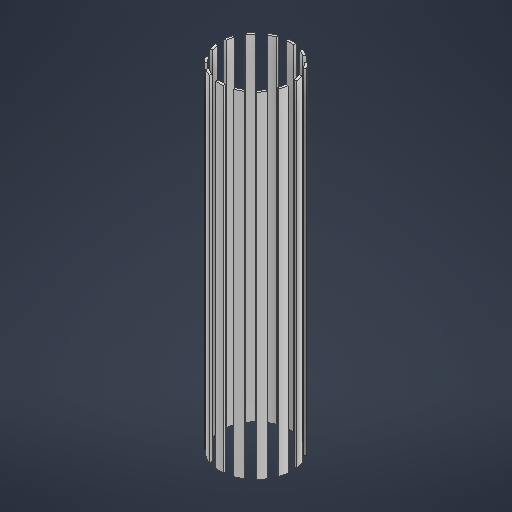
# Autodesk Inventor part: bandspreroller
Saved by Autodesk Inventor 2026.1 (Build 301233000, 233)
## iProperties
Created: 2025-08-08
Part Number: bandspreroller
Material: Generic
Document SubType Name: Modeling
Designer: roejo
Density: 1 g/cm^3
Appearance: Default
Author: roejo
Autodesk Inventor part; units mm, degrees
ref_plane "YZ Plane" through (0, 0, 0) normal (1, 0, 0) x (0, 1, 0)
ref_plane "XZ Plane" through (0, 0, 0) normal (0, 1, 0) x (-1, 0, 0)
ref_plane "XY Plane" through (0, 0, 0) normal (0, 0, 1) x (1, 0, 0)
sketch "Sketch1" plane through (0, 0, 0) normal (0, 1, 0) x (-1, 0, 0)
  circle A0 centre (0, 0) radius 24.4475
  dimension "d0" = 48.895
  constraints: 1 centre point, 1 coincident
  measures "d0" diameter of A0
extrude "Extrusion1" add sketch "Sketch1" along normal blind 224.3328
sketch "Sketch2" plane through (0, 224.3328, 0) normal (0, 1, 0) x (1, 0, 0)
  circle A0 centre (0, 0) radius 22.86
  dimension "d3" = 45.72
  constraints: 1 centre point, 1 coincident
  measures "d3" diameter of A0
extrude "Extrusion2" cut sketch "Sketch2" against normal through all
sketch "Sketch3" plane through (0, 224.3328, 0) normal (0, 1, 0) x (1, 0, 0)
  line L0 (-25.4, -2.8575) -> (-12.7, -2.8575)
  line L1 (-12.7, -2.8575) -> (-12.7, 2.8575)
  line L2 (-12.7, 2.8575) -> (-25.4, 2.8575)
  line L3 (-25.4, 2.8575) -> (-25.4, -2.8575)
  line L4 (-21.6448, -13.5952) -> (-10.2025, -8.0848)
  line L5 (-10.2025, -8.0848) -> (-12.6821, -2.9358)
  line L6 (-12.6821, -2.9358) -> (-24.1244, -8.4461)
  line L7 (-24.1244, -8.4461) -> (-21.6448, -13.5952)
  line L8 (-13.6026, -21.6401) -> (-5.6842, -11.7109)
  line L9 (-5.6842, -11.7109) -> (-10.1524, -8.1476)
  line L10 (-10.1524, -8.1476) -> (-18.0707, -18.0769)
  line L11 (-18.0707, -18.0769) -> (-13.6026, -21.6401)
  line L12 (-2.8662, -25.399) -> (-0.0402, -13.0174)
  line L13 (-0.0402, -13.0174) -> (-5.6119, -11.7457)
  line L14 (-5.6119, -11.7457) -> (-8.4379, -24.1273)
  line L15 (-8.4379, -24.1273) -> (-2.8662, -25.399)
  line L16 (8.4379, -24.1273) -> (5.6119, -11.7457)
  line L17 (5.6119, -11.7457) -> (0.0402, -13.0174)
  line L18 (0.0402, -13.0174) -> (2.8662, -25.399)
  line L19 (2.8662, -25.399) -> (8.4379, -24.1273)
  line L20 (18.0707, -18.0769) -> (10.1524, -8.1476)
  line L21 (10.1524, -8.1476) -> (5.6842, -11.7109)
  line L22 (5.6842, -11.7109) -> (13.6026, -21.6401)
  line L23 (13.6026, -21.6401) -> (18.0707, -18.0769)
  line L24 (24.1244, -8.4461) -> (12.6821, -2.9358)
  line L25 (12.6821, -2.9358) -> (10.2025, -8.0848)
  line L26 (10.2025, -8.0848) -> (21.6448, -13.5952)
  line L27 (21.6448, -13.5952) -> (24.1244, -8.4461)
  line L28 (25.4, 2.8575) -> (12.7, 2.8575)
  line L29 (12.7, 2.8575) -> (12.7, -2.8575)
  line L30 (12.7, -2.8575) -> (25.4, -2.8575)
  line L31 (25.4, -2.8575) -> (25.4, 2.8575)
  circle A0 centre (0, 0) radius 24.4475 projected
  line L32 (21.6448, 13.5952) -> (10.2025, 8.0848)
  line L33 (10.2025, 8.0848) -> (12.6821, 2.9358)
  line L34 (12.6821, 2.9358) -> (24.1244, 8.4461)
  line L35 (24.1244, 8.4461) -> (21.6448, 13.5952)
  line L36 (13.6026, 21.6401) -> (5.6842, 11.7109)
  line L37 (5.6842, 11.7109) -> (10.1524, 8.1476)
  line L38 (10.1524, 8.1476) -> (18.0707, 18.0769)
  line L39 (18.0707, 18.0769) -> (13.6026, 21.6401)
  line L40 (2.8662, 25.399) -> (0.0402, 13.0174)
  line L41 (0.0402, 13.0174) -> (5.6119, 11.7457)
  line L42 (5.6119, 11.7457) -> (8.4379, 24.1273)
  line L43 (8.4379, 24.1273) -> (2.8662, 25.399)
  line L44 (-8.4379, 24.1273) -> (-5.6119, 11.7457)
  line L45 (-5.6119, 11.7457) -> (-0.0402, 13.0174)
  line L46 (-0.0402, 13.0174) -> (-2.8662, 25.399)
  line L47 (-2.8662, 25.399) -> (-8.4379, 24.1273)
  line L48 (-18.0707, 18.0769) -> (-10.1524, 8.1476)
  line L49 (-10.1524, 8.1476) -> (-5.6842, 11.7109)
  line L50 (-5.6842, 11.7109) -> (-13.6026, 21.6401)
  line L51 (-13.6026, 21.6401) -> (-18.0707, 18.0769)
  line L52 (-24.1244, 8.4461) -> (-12.6821, 2.9358)
  line L53 (-12.6821, 2.9358) -> (-10.2025, 8.0848)
  line L54 (-10.2025, 8.0848) -> (-21.6448, 13.5952)
  line L55 (-21.6448, 13.5952) -> (-24.1244, 8.4461)
  point P0 (-30.1625, 0)
  point P1 (-27.1755, -13.087)
  point P2 (-18.806, -23.582)
  point P3 (-6.7118, -29.4063)
  point P4 (6.7118, -29.4063)
  point P5 (18.806, -23.582)
  point P6 (27.1755, -13.087)
  point P7 (30.1625, 0)
  point P8 (27.1755, 13.087)
  point P9 (18.806, 23.582)
  point P10 (6.7118, 29.4063)
  point P11 (-6.7118, 29.4063)
  point P12 (-18.806, 23.582)
  point P13 (-27.1755, 13.087)
  dimension "d13" = 360
  dimension "d16" = 12.7
  constraints: 112 end point, 2 parallel, 1 horizontal, 1 perpendicular, 127 other
  measures "d16" distance from line of A0.centre L1
extrude "Extrusion3" cut sketch "Sketch3" against normal through all contours L3 L2 A0 L0 | A0 L2 L1 L0 | A0 L4 L7 L6 | L6 L5 L4 A0 | L52 L55 L54 A0 | A0 L54 L53 L52 | A0 L8 L11 L10 | L10 L9 L8 A0 | L48 L51 L50 A0 | A0 L50 L49 L48 | A0 L12 L15 L14 | L14 L13 L12 A0 | L44 L47 L46 A0 | A0 L46 L45 L44 | A0 L16 L19 L18 | L18 L17 L16 A0 | L40 L43 L42 A0 | A0 L42 L41 L40 | A0 L20 L23 L22 | L22 L21 L20 A0 | L36 L39 L38 A0 | A0 L38 L37 L36 | A0 L24 L27 L26 | L26 L25 L24 A0 | L32 L35 L34 A0 | A0 L34 L33 L32 | A0 L28 L31 L30 | L30 L29 L28 A0
body "Solid1"
